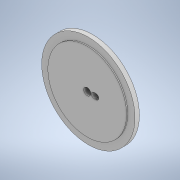
# Autodesk Inventor part: Deckel
Saved by Autodesk Inventor 2021 (Build 250183000, 183)
## iProperties
Created: 2021-05-17
Part Number: Deckel
Material: Generic
Document SubType Name: Modeling
Designer: Timo
Density: 1 g/cm^3
Appearance: Default
Author: Timo
Autodesk Inventor part; units mm, degrees
ref_plane "YZ Plane" through (0, 0, 0) normal (1, 0, 0) x (0, 1, 0)
ref_plane "XZ Plane" through (0, 0, 0) normal (0, 1, 0) x (-1, 0, 0)
ref_plane "XY Plane" through (0, 0, 0) normal (0, 0, 1) x (1, 0, 0)
sketch "Sketch1" plane through (0, 0, 0) normal (0, 0, 1) x (1, 0, 0)
  circle A0 centre (0, 0) radius 85
  dimension "d0" = 170
  constraints: 1 centre point, 1 coincident
  measures "d0" diameter of A0
extrude "Extrusion1" add sketch "Sketch1" along normal blind 8
sketch "Sketch2" plane through (0, 0, 8) normal (0, 0, 1) x (1, 0, 0)
  circle A0 centre (0, 0) radius 71.75
  dimension "d3" = 143.5
  constraints: 1 centre point, 1 coincident
  measures "d3" diameter of A0
extrude "Extrusion2" add sketch "Sketch2" along normal blind 2
sketch "Sketch3" plane through (0, 0, 10) normal (0, 0, 1) x (1, 0, 0)
  circle A0 centre (0, 0) radius 6.5
  dimension "d6" = 13
  constraints: 1 centre point, 1 coincident
  measures "d6" diameter of A0
extrude "Extrusion3" cut sketch "Sketch3" against normal through all
sketch "Sketch4" plane through (0, 0, 0) normal (0, 1, 0) x (-1, 0, 0)
  line L0 (0, 53) -> (-39.9771, -56.8361) construction
  line L1 (85, 8) -> (-85, 8) construction
  line L2 (0, -78.8034) -> (0, 74.9672) construction
  point P0 (0, 0)
  dimension "d9" = 45
  dimension "d10" = 20
  constraints: 2 end point, 1 point on line
  measures "d9" distance from line of L0.start L1
  measures "d10" angle of L2 L0
ref_plane "Work Plane1" through (19.2904, 0, 0) normal (0.3420201, 0, -0.9396926) x (0, 1, 0)
sketch "Sketch5" plane through (19.2904, 0, 0) normal (0.3420201, 0, -0.9396926) x (0, 1, 0)
  line L0 (0, 0) -> (0, -2.8191) construction
  line L1 (-5, 0) -> (-5, -2.8191)
  line L2 (5, -2.8191) -> (5, 0)
  arc A0 (5, 0) -> (-5, 0) centre (0, 0) ccw
  arc A1 (-5, -2.8191) -> (5, -2.8191) centre (0, -2.8191) ccw
  line L3 (0, 0) -> (0, -2) construction
  line L4 (-5, 0) -> (-5, -2)
  line L5 (5, -2) -> (5, 0)
  arc A2 (5, 0) -> (-5, 0) centre (0, 0) ccw
  arc A3 (-5, -2) -> (5, -2) centre (0, -2) ccw
  point P0 (0, -18.1271)
  point P1 (0, -1.4095)
  point P2 (0, -1)
  point P3 (-5, -2)
  point P4 (5, -2)
  dimension "d12" = 10
  dimension "d13" = 2.8191
  dimension "d37" = 2
  constraints: 16 end point, 8 point on circle, 8 tangent, 4 centre point, 2 midpoint, 2 parallel, 1 coincident, 1 point on line, 1 vertical
  measures "d12" diameter of A1
  measures "d13" distance of L0.end L0.start
  measures "d37" distance of L0.start L3.end
extrude "Extrusion4" cut sketch "Sketch5" against normal through all both and the other way through all
sketch "Sketch10" plane through (0, 0, 0) normal (0, 0, -1) x (-1, 0, 0)
  line L0 (119, 0) -> (-119, 0) projected
  line L1 (0, 0) -> (-18.2904, -11.65) construction
  line L2 (-18.2904, -11.65) -> (-18.2904, -5) construction
  line L3 (-16.2904, -5) -> (-19.2904, -5) construction
  point P0 (-18.2904, 11.65)
  point P1 (-30, 0)
  dimension "d50" = 30
  dimension "d60" = 11.65
  dimension "d61" = 1
  constraints: 4 end point, 2 point on line, 1 symmetric about line, 1 vertical
  measures "d50" distance of L1.start point (-30, 0)
  measures "d60" distance from line of L0 L1.end
  measures "d61" distance from line of L3.end L2
hole "Hole1" at (18.2904, -11.65, 0) at (18.2904, 11.65, 0) at (30, 0, 0) direction (0, 0, 1) diameter 2.459 depth 6 tip angle 118 thread size "M3x0.5" class "6H" standard "ANSI Metric M Profile"
body "Solid1"
